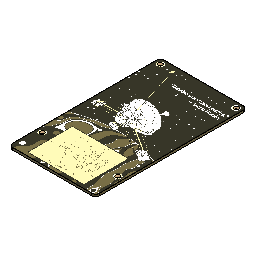
5128 MacroPad RP2040-bottom-plate (Autodesk Fusion 360 design; units mm, degrees)
part number: MOUNTINGHOLE3.0THIN
Autodesk Fusion 360 part; units mm, degrees
sketch "sketch 306" plane through (0, 0, 0) normal (0, 0, 1) x (1, 0, 0)
  line L0 (0, 101.6) -> (0, 2.54)
  arc A0 (0, 2.54) -> (2.54, 0) centre (2.54, 2.54) ccw
  line L1 (2.54, 0) -> (57.15, 0)
  arc A1 (57.15, 0) -> (59.69, 2.54) centre (57.15, 2.54) ccw
  line L2 (59.69, 2.54) -> (59.69, 101.6)
  arc A2 (59.69, 101.6) -> (57.15, 104.14) centre (57.15, 101.6) ccw
  line L3 (57.15, 104.14) -> (2.54, 104.14)
  arc A3 (2.54, 104.14) -> (0, 101.6) centre (2.54, 101.6) ccw
extrude "Board" add sketch "sketch 306" along normal blind 1.57 makes body 1 in component "Board"
sketch "sketch 604" plane through (0, 0, 0) normal (0, 0, 1) x (1, 0, 0)
  line L0 (-2.2, -2.2) -> (2.2, -2.2)
  line L1 (2.2, -2.2) -> (2.2, 2.2)
  line L2 (2.2, 2.2) -> (-2.2, 2.2)
  line L3 (-2.2, 2.2) -> (-2.2, -2.2)
extrude "MOUNTINGHOLE_3.0_PLATEDTHIN" add sketch "sketch 604" along normal blind 0.1 separate body makes body 2 in component "MOUNTINGHOLE_3.0_PLATEDTHIN"
sketch "sketch 739" plane through (0, 0, 0) normal (0, 0, 1) x (1, 0, 0)
  line L0 (-0.01, -0.011) -> (59.68, -0.011)
  line L1 (59.68, -0.011) -> (59.68, 104.129)
  line L2 (59.68, 104.129) -> (-0.01, 104.129)
  line L3 (-0.01, 104.129) -> (-0.01, -0.011)
extrude "MACROPAD_BACKPLATE_FRONT" add sketch "sketch 739" along normal blind 0.1 separate body makes body 3 in component "MACROPAD_BACKPLATE_FRONT"
sketch "sketch 874" plane through (0, 0, 0) normal (0, 0, 1) x (1, 0, 0)
  line L0 (0.478, 0.476) -> (59.192, 0.476)
  line L1 (59.192, 0.476) -> (59.192, 103.643)
  line L2 (59.192, 103.643) -> (0.478, 103.643)
  line L3 (0.478, 103.643) -> (0.478, 0.476)
extrude "MACROPAD_BACKPLATE_BACK" add sketch "sketch 874" along normal blind 0.1 separate body makes body 4 in component "MACROPAD_BACKPLATE_BACK"
sketch "sketch 1177" plane through (0, 0, 0) normal (0, 0, 1) x (1, 0, 0)
  circle A0 centre (3.81, 19.05) radius 1.5
  circle A1 centre (55.88, 19.05) radius 1.5
  circle A2 centre (3.81, 100.33) radius 1.5
  circle A3 centre (55.88, 100.33) radius 1.5
extrude "Extrude4" cut sketch "sketch 1177" along normal blind 1.57 bodies 1 in component "Board"
component "PCB Component" placed x (1, 0, 0) y (0, 1, 0) z (0, 0, 1) at (0, 0, 0)
component "Board" placed x (1, 0, 0) y (0, 1, 0) z (0, 0, 1) at (0, 0, 0) in component "PCB Component"
component "MOUNTINGHOLE_3.0_PLATEDTHIN" placed x (1, 0, 0) y (0, 1, 0) z (0, 0, 1) at (3.81, 19.05, 1.57) in component "PCB Component"
component "MOUNTINGHOLE_3.0_PLATEDTHIN" placed x (1, 0, 0) y (0, 1, 0) z (0, 0, 1) at (55.88, 19.05, 1.57) in component "PCB Component"
component "MOUNTINGHOLE_3.0_PLATEDTHIN" placed x (1, 0, 0) y (0, 1, 0) z (0, 0, 1) at (3.81, 100.33, 1.57) in component "PCB Component"
component "MOUNTINGHOLE_3.0_PLATEDTHIN" placed x (1, 0, 0) y (0, 1, 0) z (0, 0, 1) at (55.88, 100.33, 1.57) in component "PCB Component"
component "MACROPAD_BACKPLATE_FRONT" placed x (-1, 0, 0) y (0, 1, 0) z (0, 0, -1) at (59.69, 0, 0) in component "PCB Component"
component "MACROPAD_BACKPLATE_BACK" placed x (1, 0, 0) y (0, 1, 0) z (0, 0, 1) at (0, 0, 1.57) in component "PCB Component"
named bodies: "Board", "MOUNTINGHOLE_3.0_PLATEDTHIN", "MACROPAD_BACKPLATE_FRONT", "MACROPAD_BACKPLATE_BACK"
